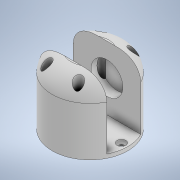
# Autodesk Inventor part: tilt_1_base
Saved by Autodesk Inventor 2022.3 (Build 263350000, 350)
## iProperties
Created: 2022-05-28
Part Number: tilt_1_base
Material: Generic
Document SubType Name: Modeling
Designer: Mlees
Density: 1 g/cm^3
Appearance: Default
Author: Mlees
Autodesk Inventor part; units mm, degrees
ref_plane "YZ Plane" through (0, 0, 0) normal (1, 0, 0) x (0, 1, 0)
ref_plane "XZ Plane" through (0, 0, 0) normal (0, 1, 0) x (-1, 0, 0)
ref_plane "XY Plane" through (0, 0, 0) normal (0, 0, 1) x (1, 0, 0)
sketch "Sketch1" plane through (0, 0, 0) normal (0, 1, 0) x (-1, 0, 0)
  circle A0 centre (0, 0) radius 30
  circle A1 centre (-25, 0) radius 1.5
  circle A2 centre (-12.5, -21.6506) radius 1.5
  circle A3 centre (12.5, -21.6506) radius 1.5
  circle A4 centre (25, 0) radius 1.5
  circle A5 centre (12.5, 21.6506) radius 1.5
  circle A6 centre (-12.5, 21.6506) radius 1.5
  dimension "d0" = 60
  dimension "d2" = 3
  dimension "d5" = 360
  constraints: 7 centre point, 1 coincident, 13 other
  measures "d0" diameter of A0
  measures "d2" diameter of A1
extrude "Extrusion1" add sketch "Sketch1" along normal blind 3
fillet "Fillet1" radius 2 6 edges at (-11, 3, 21.6506) (-23.5, 3, 0) (-11, 3, -21.6506) (14, 3, -21.6506) (26.5, 3, 0) (14, 3, 21.6506) inverted yes
sketch "Sketch5" plane through (0, 3, 0) normal (0, 1, 0) x (1, 0, 0)
  circle A0 centre (0, 0) radius 30
  constraints: 1 centre point, 1 coincident
extrude "Extrusion5" add sketch "Sketch5" along normal blind 50.8
fillet "Fillet3" radius 15 1 edges at (-30, 53.8, 0)
sketch "Sketch6" plane through (0, 53.8, 0) normal (0, 1, 0) x (1, 0, 0)
  circle A0 centre (-25, 0) radius 1.5 projected
  circle A1 centre (-25, 0) radius 3.5
  circle A2 centre (0, 0) radius 15
  circle A3 centre (-12.5, -21.6506) radius 3.5
  circle A4 centre (12.5, -21.6506) radius 3.5
  circle A5 centre (25, 0) radius 3.5
  circle A6 centre (12.5, 21.6506) radius 3.5
  circle A7 centre (-12.5, 21.6506) radius 3.5
  dimension "d29" = 360
  constraints: 7 centre point, 2 coincident, 13 other
extrude "Extrusion6" cut sketch "Sketch6" against normal blind 50.8 contours A0 | A1 | A3 | A4 | A5 | A6 | A7
sketch "Sketch7" plane through (0, 53.8, 0) normal (0, 1, 0) x (1, 0, 0)
  line L0 (-23, 13.5) -> (26.7909, 13.5)
  circle A0 centre (0, 0) radius 30 projected
  line L1 (-23, 13.5) -> (-26.7909, 13.5)
  line L2 (0, 0) -> (-7.0863, 0)
  line L3 (-23, -13.5) -> (26.7909, -13.5)
  line L4 (-23, -13.5) -> (-26.7909, -13.5)
  arc A1 (-26.7909, 13.5) -> (-26.7909, -13.5) centre (0, 0) ccw
  arc A2 (26.7909, -13.5) -> (26.7909, 13.5) centre (0, 0) ccw
  point P0 (26.7909, -13.5)
  constraints: 10 end point, 6 point on circle, 3 symmetric about line, 2 centre point, 2 concentric, 2 horizontal
extrude "Extrusion7" cut sketch "Sketch7" against normal blind 50.8 contours L0 A0 L3 L4 L1
ref_plane "Work Plane1" through (-6.5383, 53.8, 0) normal (0, 0, 1) x (1, 0, 0)
sketch "Sketch8" plane through (-6.5383, 53.8, -13.5) normal (0, 0, 1) x (1, 0, 0)
  line L0 (0, 0) -> (13.0767, 0) projected
  line L1 (-20.2525, -50.8) -> (33.3292, -50.8) projected
  circle A0 centre (6.5383, -25.4) radius 12.625
  point P0 (6.5383, -53.8)
  dimension "d38" = 25.25
  constraints: 1 centre point
  measures "d38" diameter of A0
extrude "Extrusion8" cut sketch "Sketch8" against normal blind 8
body "Solid1"
